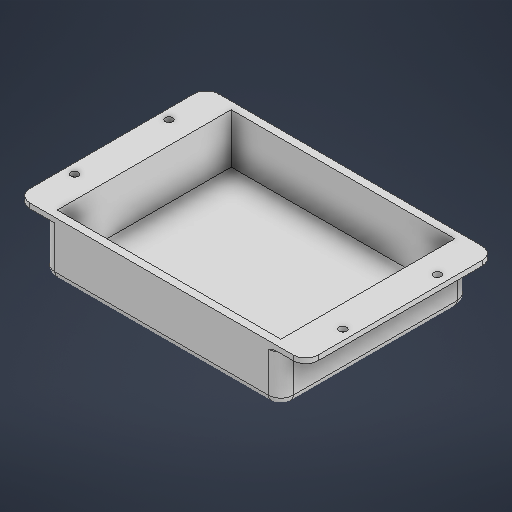
# Autodesk Inventor part: battary holder
Saved by Autodesk Inventor 2026.1 (Build 301233000, 233)
## iProperties
Created: 2026-03-06
Part Number: battary holder
Material: Generic
Document SubType Name: Modeling
Designer: momen
Density: 1 g/cm^3
Appearance: Default
Author: momen
Autodesk Inventor part; units mm, degrees
ref_plane "YZ Plane" through (0, 0, 0) normal (1, 0, 0) x (0, 1, 0)
ref_plane "XZ Plane" through (0, 0, 0) normal (0, 1, 0) x (-1, 0, 0)
ref_plane "XY Plane" through (0, 0, 0) normal (0, 0, 1) x (1, 0, 0)
sketch "Sketch1" plane through (0, 0, 0) normal (0, 1, 0) x (-1, 0, 0)
  line L0 (-45, 35) -> (45, 35)
  line L1 (45, 35) -> (45, -35)
  line L2 (45, -35) -> (-45, -35)
  line L3 (-45, -35) -> (-45, 35)
  line L4 (-45, 35) -> (45, -35) construction
  line L5 (45, 35) -> (-45, -35) construction
  line L6 (-48, 38) -> (48, 38)
  line L7 (48, 38) -> (48, -38)
  line L8 (48, -38) -> (-48, -38)
  line L9 (-48, -38) -> (-48, 38)
  line L10 (-48, 38) -> (48, -38) construction
  line L11 (48, 38) -> (-48, -38) construction
  line L12 (48, 38) -> (58, 38)
  line L13 (58, 38) -> (58, -38)
  line L14 (58, -38) -> (48, -38)
  line L15 (48, -38) -> (48, 38)
  line L16 (-48, 38) -> (-58, 38)
  line L17 (-58, 38) -> (-58, -38)
  line L18 (-58, -38) -> (-48, -38)
  line L19 (-48, -38) -> (-48, 38)
  line L20 (54, -19) -> (54, 19)
  line L21 (54, -19) -> (92, -19) construction
  circle A0 centre (54, 19) radius 1.5
  circle A1 centre (54, -19) radius 1.5
  line L22 (-54, -19) -> (-54, 19)
  circle A2 centre (-54, 19) radius 1.5
  circle A3 centre (-54, -19) radius 1.5
  line L23 (58, 0) -> (54, 0)
  line L24 (-58, 0) -> (-54, 0)
  point P0 (0, 0)
  point P1 (54, 0)
  dimension "d0" = 90
  dimension "d1" = 70
  dimension "d2" = 96
  dimension "d3" = 76
  dimension "d4" = 10
  dimension "d5" = 76
  dimension "d6" = 10
  dimension "d7" = 76
  dimension "d8" = 38
  dimension "d9" = 90
  dimension "d10" = 3
  dimension "d11" = 3
  dimension "d12" = 3
  dimension "d13" = 3
  dimension "d23" = 4
  dimension "d24" = 4
  constraints: 50 end point, 9 parallel, 8 midpoint, 7 horizontal, 5 perpendicular, 4 centre point, 4 coincident, 1 vertical
  measures "d0" distance of L1.end L2.end
  measures "d1" distance of L0.end L1.end
  measures "d2" distance of L7.end L8.end
  measures "d3" distance of L6.end L7.end
  measures "d4" distance of L13.end L14.end
  measures "d5" distance of L12.end L13.end
  measures "d6" distance of L18.end L17.end
  measures "d7" distance of L17.end L16.end
  measures "d8" distance of L20.start L20.end
  measures "d9" angle of L21 L20
  measures "d10" diameter of A0
  measures "d11" diameter of A1
  measures "d12" diameter of A2
  measures "d13" diameter of A3
  measures "d23" distance of L23.start L23.end
  measures "d24" distance of L24.start L24.end
extrude "Extrusion1" add sketch "Sketch1" against normal blind 20 contours L6 L7 L8 L9
extrude "Extrusion2" add sketch "Sketch1" against normal blind 2 contours L9 L18 L17 L16 | L12 L13 L14 L7
sketch "Sketch2" plane through (0, -20, 0) normal (0, -1, 0) x (1, 0, 0)
  line L0 (-48, -38) -> (48, -38) projected
  line L1 (-48, 38) -> (48, 38)
  line L2 (48, 38) -> (48, -38)
  line L3 (48, -38) -> (-48, -38)
  line L4 (-48, -38) -> (-48, 38)
  line L5 (-48, 38) -> (48, -38) construction
  line L6 (48, 38) -> (-48, -38) construction
  point P0 (0, 0)
  constraints: 12 end point, 2 midpoint, 2 parallel, 1 horizontal, 1 perpendicular
extrude "Extrusion3" add sketch "Sketch2" along normal blind 2
fillet "Fillet1" radius 5 8 edges at (48, -12, -38) (-48, -12, -38) (48, -12, 38) (-48, -12, 38) (-58, -1, 38) (-58, -1, -38) (58, -1, -38) (58, -1, 38)
fillet "Fillet2" radius 1 1 edges at (48, -2, 0)
fillet "Fillet3" radius 3 8 edges at (-46.5355, -22, 36.5355) (-48, -22, 0) (-46.5355, -22, -36.5355) (0, -22, -38) (46.5355, -22, -36.5355) (48, -22, 0) (46.5355, -22, 36.5355) (0, -22, 38)
body "Solid1"
